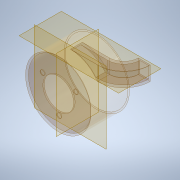
# Autodesk Inventor part: Dust Bin
Saved by Autodesk Inventor 2020 (Build 240168000, 168)
## iProperties
Created: 2020-03-28
Part Number: Dust Bin
Material: Generic
Document SubType Name: Modeling
Designer: pengpeng
Density: 1 g/cm^3
Appearance: Polycarbonate - Smoked
Author: pengpeng
Autodesk Inventor part; units mm, degrees
ref_plane "XY Plane" through (0, 0, 0) normal (0, 0, 1) x (1, 0, 0)
sketch "Sketch1" plane through (0, 0, 0) normal (0, 0, 1) x (1, 0, 0)
  circle A0 centre (0, 0) radius 68
  dimension "d1" = 136
  constraints: 1 centre point
  measures "d1" diameter of A0
extrude "Extrusion1" add sketch "Sketch1" along normal blind 80
shell "Shell1" thickness 3 removed faces 1 at (13.6377, 7.7647, 0)
sketch "Sketch2" plane through (0, 0, 80) normal (0, 0, 1) x (1, 0, 0)
  circle A0 centre (0, 0) radius 32
  dimension "d5" = 64
  constraints: 1 centre point, 1 coincident
  measures "d5" diameter of A0
extrude "Extrusion2" cut sketch "Sketch2" against normal up to surface (3 mm away)
sketch "Sketch3" plane through (0, 0, 77) normal (0, 0, -1) x (-1, 0, 0)
  circle A0 centre (0, 0) radius 32 projected
  circle A1 centre (0, 0) radius 65 projected
  circle A2 centre (0, -40) radius 4.8
  line L0 (0, 0) -> (0, -56.282) construction
  line L1 (0, 0) -> (-47.9956, 27.7103) construction
  line L2 (0, 0) -> (60.1339, 34.7183) construction
  circle A3 centre (-34.641, 20) radius 4.8
  circle A4 centre (34.641, 20) radius 4.8
  dimension "d8" = 9.6
  dimension "d9" = 40
  dimension "d10" = 120
  dimension "d11" = 120
  dimension "d12" = 9.6
  dimension "d13" = 9.6
  dimension "d14" = 40
  dimension "d15" = 40
  constraints: 6 end point, 3 centre point, 2 point on line, 1 vertical
  measures "d8" diameter of A2
  measures "d9" distance of point (0, 0) A2.centre
  measures "d10" angle of L0 L1
  measures "d11" angle of L0 L2
  measures "d12" diameter of A3
  measures "d13" diameter of A4
  measures "d14" distance of point (0, 0) A4.centre
  measures "d15" distance of point (0, 0) A3.centre
extrude "Extrusion3" cut sketch "Sketch3" against normal blind 1.524 contours A2 | A3 | A4
ref_plane "Work Plane1" through (0, 0, 55) normal (0, 0, 1) x (1, 0, 0)
sketch "Sketch4" plane through (0, 0, 55) normal (0, 0, 1) x (1, 0, 0)
  circle A0 centre (0, 0) radius 68 projected
  circle A1 centre (0, 0) radius 68 projected
  line L0 (0, 68) -> (56.3915, 68)
  line L1 (56.3915, 68) -> (56.3915, 38)
  line L2 (56.3915, 38) -> (0, 38)
  line L3 (0, 38) -> (0, 68)
  dimension "d24" = 30
  constraints: 8 end point, 2 horizontal, 2 parallel, 1 perpendicular, 1 vertical alignment, 3 other
  measures "d24" distance between parallel lines of L2 L0
extrude "Extrusion4" add sketch "Sketch4" against normal blind 25 contours A0 L0 L1
sketch "Sketch6" plane through (56.3915, 38, 55) normal (1, 0, 0) x (0, 0, -1)
  line L0 (0, 0) -> (0, 30) projected
  line L1 (25, 0) -> (0, 0) projected
  line L2 (25, 30) -> (25, 0) projected
  line L3 (0, 30) -> (25, 30) projected
  line L4 (22, 27) -> (22, 3)
  line L5 (22, 3) -> (3, 3)
  line L6 (3, 3) -> (3, 27)
  line L7 (3, 27) -> (22, 27)
  point P0 (55, -38)
  dimension "d27" = 3
  constraints: 8 end point, 3 other
  measures "d27" distance between parallel lines of L3 L7
extrude "Extrusion5" cut sketch "Sketch6" against normal blind 56.391 contours L4 L5 L6 L7
ref_plane "Work Plane4" through (0, 68, 0) normal (0, 1, 0) x (-1, 0, 0)
sketch "Sketch9" plane through (56.3915, 38, 55) normal (1, 0, 0) x (0, 0, -1)
  line L0 (3, 3) -> (3, 27) projected
  line L1 (3, 27) -> (22, 27) projected
  line L2 (22, 27) -> (22, 3) projected
  line L3 (22, 3) -> (3, 3) projected
  line L4 (0, 0) -> (0, 30) projected
  line L5 (25, 0) -> (0, 0) projected
  line L6 (25, 30) -> (25, 0) projected
  line L7 (0, 30) -> (25, 30) projected
  point P0 (55, -38)
sketch "Sketch10" plane through (0, 68, 0) normal (0, 1, 0) x (-1, 0, 0)
  circle A0 centre (-56.3915, 0) radius 55 construction
  line L0 (-127.7058, 55) -> (100.6176, 55) projected
  line L1 (-56.3915, 55) -> (0, 55) projected
  line L2 (0, 0) -> (-96.3915, 0) construction
  arc A1 (-56.3915, 55) -> (-111.3915, 0) centre (-56.3915, 0) ccw
  constraints: 4 point on circle, 2 centre point, 2 coincident, 2 end point, 1 horizontal, 1 point on line, 1 tangent
sweep "Sweep2" add profiles "Sketch9" path "Sketch10" path curves A1
equation "\"d11\" = d10"
equation "\"d12\" = d8"
equation "\"d13\" = d8"
equation "\"d14\" = d9"
equation "\"d15\" = d9"
body "Solid1"
